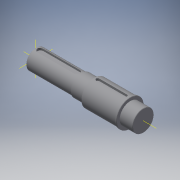
# Autodesk Inventor part: GonjenoVratilo
Saved by Autodesk Inventor 2018 (Build 220112000, 112)
## iProperties
Created: 2018-11-17
Part Number: GonjenoVratilo
Material: Generic
Document SubType Name: Modeling
Designer: Kristijan
Density: 1 g/cm^3
Appearance: Default
Author: Kristijan
Autodesk Inventor part; units mm, degrees
ref_plane "YZ Plane" through (0, 0, 0) normal (1, 0, 0) x (0, 1, 0)
ref_plane "XY Plane" through (0, 0, 0) normal (0, 0, 1) x (1, 0, 0)
sketch "Sketch1" plane through (0, 0, 0) normal (0, 0, 1) x (1, 0, 0)
  point P0 (0, 0)
sketch "Sketch2" plane through (0, 0, 0) normal (0, 0, 1) x (1, 0, 0)
  line L0 (0, 0) -> (0, 29)
  line L1 (1, 30) -> (140, 30)
  line L2 (140, 30) -> (140, 32.5)
  line L3 (140, 32.5) -> (175, 32.5)
  line L4 (180, 37.5) -> (180, 40)
  line L5 (180, 40) -> (285, 40)
  line L6 (285, 40) -> (285, 42)
  line L7 (285, 42) -> (290, 42)
  line L8 (290, 42) -> (290, 37.5)
  line L9 (300, 32.5) -> (329, 32.5)
  line L10 (330, 31.5) -> (330, 0)
  line L11 (330, 0) -> (0, 0)
  line L12 (0, 29) -> (1, 30)
  line L13 (329, 32.5) -> (330, 31.5)
  line L14 (-66, 0) -> (396, 0) projected
  line L15 (290, 37.5) -> (290, 32.5)
  line L16 (290, 32.5) -> (300, 32.5)
  line L17 (180, 37.5) -> (180, 32.5)
  line L18 (180, 32.5) -> (175, 32.5)
  point P0 (0, 30)
  point P1 (330, 32.5)
  dimension "d0" = 30
  dimension "d1" = 140
  dimension "d2" = 32.5
  dimension "d3" = 40
  dimension "d4" = 105
  dimension "d5" = 5
  dimension "d6" = 40
  dimension "d7" = 32.5
  dimension "d8" = 40
  dimension "d9" = 2
  dimension "d10" = 1
  dimension "d11" = 45
  dimension "d12" = 1
  dimension "d13" = 45
  constraints: 36 end point, 11 perpendicular, 8 point on line, 4 vertical, 1 horizontal
  measures "d0" distance between parallel lines of L11 L1
  measures "d1" distance of point (0, 30) L1.end
  measures "d2" distance between parallel lines of L11 L3
  measures "d3" distance of L2.end L17.end
  measures "d4" distance of L4.end L5.end
  measures "d5" distance of L6.end L7.end
  measures "d6" distance of L15.end point (330, 32.5)
  measures "d7" distance between parallel lines of L11 L9
  measures "d8" distance between parallel lines of L11 L5
  measures "d9" distance of L5.end L6.end
  measures "d10" distance of L0.end point (0, 30)
  measures "d11" angle of L0 L12
  measures "d12" distance of L9.end point (330, 32.5)
  measures "d13" angle of L9 L13
revolve "Revolution1" add sketch "Sketch2" angle 360 about axis through (-10, 0, 0) along (1, 0, 0)
ref_plane "Work Plane1" through (70.5, 30, 0) normal (0, 1, 0) x (-1, 0, 0)
ref_plane "Work Plane2" through (232.5, 40, 0) normal (0, 1, 0) x (-1, 0, 0)
sketch "Sketch3" plane through (70.5, 30, 0) normal (0, 1, 0) x (-1, 0, 0)
  line L0 (56.5, 0) -> (-55.5, 0) construction
  line L1 (56.5, 9) -> (-55.5, 9)
  line L2 (-55.5, -9) -> (56.5, -9)
  arc A0 (56.5, -9) -> (56.5, 9) centre (56.5, 0) ccw
  arc A1 (-55.5, 9) -> (-55.5, -9) centre (-55.5, 0) ccw
  line L3 (-69.5, 32.5) -> (-69.5, -32.5) projected
  point P0 (70.5, 0)
  point P1 (0.5, 0)
  dimension "d16" = 130
  dimension "d17" = 5
  dimension "d18" = 9
  constraints: 8 end point, 4 point on circle, 4 tangent, 2 centre point, 1 horizontal, 1 midpoint, 1 parallel
  measures "d17" distance edge to line of A1 L3
  measures "d18" radius of A0
extrude "Extrusion1" cut sketch "Sketch3" against normal blind 7
sketch "Sketch4" plane through (232.5, 40, 0) normal (0, 1, 0) x (-1, 0, 0)
  line L0 (42.5, 0) -> (-42.5, 0) construction
  line L1 (42.5, -5) -> (-42.5, -5)
  line L2 (-42.5, 5) -> (42.5, 5)
  arc A0 (42.5, -5) -> (42.5, 5) centre (42.5, 0) ccw
  arc A1 (-42.5, 5) -> (-42.5, -5) centre (-42.5, 0) ccw
  line L3 (-52.5, 42) -> (-52.5, -42) projected
  line L4 (52.5, 40) -> (52.5, -40) projected
  point P0 (232.5, 0)
  point P1 (0, 0)
  dimension "d22" = 5
  dimension "d23" = 10
  dimension "d24" = 10
  constraints: 8 end point, 4 point on circle, 4 tangent, 2 centre point, 1 horizontal, 1 midpoint, 1 parallel
  measures "d22" radius of A0
  measures "d23" distance from line of L4 L0.start
  measures "d24" distance from line of L3 L0.end
extrude "Extrusion2" cut sketch "Sketch4" against normal blind 7
chamfer "Chamfer1" distance 1 angle 45 1 edges at (290, -42, 0) measured on face at (290, -41.5, 0)
equation "\"d6\" = d3"
equation "\"d7\" = d2"
equation "\"d12\" = d10"
equation "\"d13\" = d11"
equation "\"d24\" = d23"
body "Solid1"
